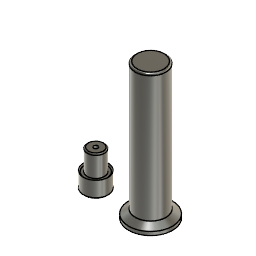
Volvo_tool_orig (Autodesk Fusion 360 design; units mm, degrees)
Autodesk Fusion 360 part; units mm, degrees
sketch "Sketch1" plane through (0, 0, 0) normal (0, 1, 0) x (1, 0, 0)
  line L0 (3.5, 0) -> (18.2, 0)
  line L1 (20.2, -2) -> (20.2, -27)
  line L2 (3.5, -60) -> (12, -60)
  line L3 (14, -58) -> (14, -25)
  line L4 (14, -25) -> (18.2, -25)
  line L5 (3.5, -60) -> (3.5, 0)
  arc A0 (20.2, -27) -> (18.2, -25) centre (18.2, -27) ccw
  arc A1 (12, -60) -> (14, -58) centre (12, -58) ccw
  arc A2 (20.2, -2) -> (18.2, 0) centre (18.2, -2) ccw
  line L6 (90, 0) -> (90, 13.6544) construction
  line L7 (110.25, 0) -> (120, 0)
  line L8 (121, -1) -> (121, -4.3)
  line L9 (121, -4.3) -> (126, -4.3)
  line L10 (126, -4.3) -> (126, -10.3)
  line L11 (126, -10.3) -> (115, -17.3)
  line L12 (115, -17.3) -> (115, -224)
  line L13 (112, -227) -> (90, -227)
  line L14 (90, -227) -> (90, -53)
  line L15 (90, -53) -> (110.25, -53)
  line L16 (110.25, -53) -> (110.25, 0)
  circle A3 centre (90, -41) radius 2.5
  arc A4 (112, -227) -> (115, -224) centre (112, -224) ccw
  arc A5 (121, -1) -> (120, 0) centre (120, -1) ccw
  point P0 (20.2, 0)
  point P1 (14, -60)
  point P2 (121, 0)
  point P3 (115, -227)
  dimension "d1" = 3.5
  dimension "d2" = 20.2
  dimension "d3" = 27
  dimension "d4" = 60
  dimension "d5" = 14
  dimension "d6" = 4
  dimension "d7" = 2
  dimension "d8" = 2
  dimension "d10" = 90
  dimension "d11" = 227
  dimension "d12" = 20.25
  dimension "d13" = 25
  dimension "d14" = 53
  dimension "d15" = 5
  dimension "d16" = 41
  dimension "d17" = 31
  dimension "d18" = 36
  dimension "d19" = 4.3
  dimension "d20" = 6
  dimension "d21" = 7
  dimension "d22" = 3
  dimension "d23" = 1
  constraint horizontal L0
  constraint perpendicular L0 L1
  constraint horizontal L2
  constraint perpendicular L2 L3
  constraint perpendicular L1 L4
  constraint vertical L5
  constraint tangent L1 A0
  constraint tangent L4 A0
  constraint horizontal origin L0.start
  constraint coincident P1 L2
  constraint coincident P1 L3
  constraint tangent L2 A1
  constraint tangent L3 A1
  constraint coincident P0 L0
  constraint coincident P0 L1
  constraint tangent L0 A2
  constraint tangent L1 A2
  constraint vertical L6
  constraint horizontal L7
  constraint perpendicular L7 L8
  constraint perpendicular L8 L9
  constraint perpendicular L9 L10
  constraint perpendicular L9 L12
  constraint perpendicular L12 L13
  constraint perpendicular L13 L14
  constraint perpendicular L14 L15
  constraint vertical L16
  constraint horizontal origin L6.start
  constraint vertical L6.start L14.end
  constraint horizontal L6.start L7.start
  constraint vertical L6.start A3.centre
  constraint coincident P3 L12
  constraint coincident P3 L13
  constraint tangent L12 A4
  constraint tangent L13 A4
  constraint coincident P2 L7
  constraint coincident P2 L8
  constraint tangent L7 A5
  constraint tangent L8 A5
  measures "d1" distance of origin L0.start
  measures "d2" distance of origin P0
  measures "d3" distance of P0 L1.end
  measures "d4" distance of L0.start L2.start
  measures "d5" horizontal distance of origin P1
  measures "d6" diameter of A0
  measures "d7" radius of A1
  measures "d8" radius of A2
  measures "d10" distance of origin L6
  measures "d11" distance of L6.start L13.end
  measures "d12" distance of L14.end L15.end
  measures "d13" distance of P3 L13.end
  measures "d14" distance of L7.start L15.end
  measures "d15" diameter of A3
  measures "d16" distance of L6.start A3.centre
  measures "d17" distance of L6.start P2
  measures "d18" horizontal distance of L6.start L9.end
  measures "d19" distance of P2 L8.end
  measures "d20" distance of L9.end L10.end
  measures "d21" vertical distance of L10.end L11.end
  measures "d22" radius of A4
  measures "d23" radius of A5
revolve "Revolve1" add sketch "Sketch1" angle 360 about axis through (0, 0, 1.75) along (0, 0, 1) contours L0 L1 L2 L3 L4 L5 A0 A1 A2 makes body 1
revolve "Revolve2" add sketch "Sketch1" angle 360 about axis through (90, 0, 0) along (0, 0, -1) separate body contours L7 L8 L9 L10 L11 L12 L13 L14 L15 L16 A4 A5 makes body 2
equation "d1 = ( 7 / 2 ) * 1 mm"
equation "d2 = ( 40.4 / 2 ) * 1 mm"
equation "d5 = ( 28 / 2 ) * 1 mm"
equation "d12 = ( 40.5 / 2 ) * 1 mm"
